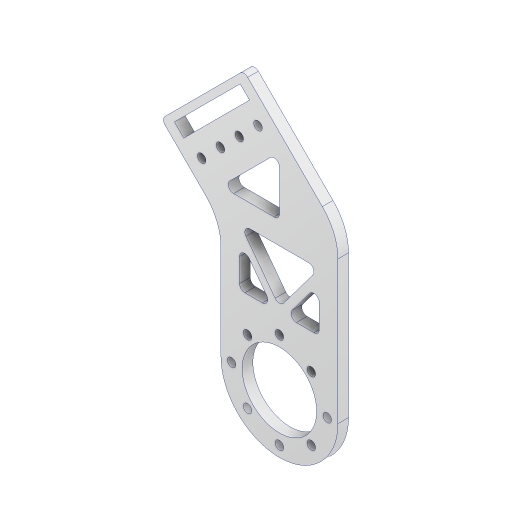
# Autodesk Inventor part: 조인트3힌지사이드_4T
Saved by Autodesk Inventor 2023.2 (Build 272271000, 271)
## iProperties
Created: 2022-01-19
Part Number: 조인트3힌지사이드_4T
Material: 알루미늄 6061
Document SubType Name: Modeling
Designer: BAEK
Density: 2.7 g/cm^3
Appearance: 알루미늄 - 평지
Mass: 34.6607 g
Surface Area: 93.0262 cm^2
Volume: 12.8373 cm^3
Author: BAEK
Autodesk Inventor part; units mm, degrees
ref_plane "YZ Plane" through (0, 0, 0) normal (1, 0, 0) x (0, 1, 0)
ref_plane "XZ Plane" through (0, 0, 0) normal (0, 1, 0) x (-1, 0, 0)
ref_plane "XY Plane" through (0, 0, 0) normal (0, 0, 1) x (1, 0, 0)
sketch "스케치1" plane through (0, 0, 0) normal (0, 0, 1) x (1, 0, 0)
  circle A0 centre (0, 0) radius 22
  line L0 (0, 0) -> (0, 18)
  line L1 (-0.15, -20.7995) -> (-0.15, -19.593)
  arc A1 (-0.15, -16.407) -> (-0.15, -19.593) centre (0, -18) ccw
  line L2 (-0.15, -16.407) -> (-0.15, -12.9991)
  arc A2 (0.15, -12.9991) -> (-0.15, -12.9991) centre (0, 0) ccw
  line L3 (0.15, -16.407) -> (0.15, -12.9991)
  arc A3 (0.15, -19.593) -> (0.15, -16.407) centre (0, -18) ccw
  line L4 (0.15, -20.7995) -> (0.15, -19.593)
  circle A4 centre (12, 12) radius 1.6
  circle A5 centre (-18, 0) radius 1.6
  circle A6 centre (-12, 12) radius 1.6
  circle A7 centre (-12, -12) radius 1.6
  circle A8 centre (18, 0) radius 1.6
  circle A9 centre (12, -12) radius 1.6
  circle A10 centre (0, 18) radius 1.6
  circle A11 centre (0, 0) radius 12.5
  circle A12 centre (0, -18) radius 1.6
  point P0 (0.15, -19.593)
  dimension "d0" = 44
  dimension "d1" = 18
  constraints: 13 centre point, 10 end point, 6 point on circle, 2 coincident, 1 concentric, 1 vertical
  measures "d0" diameter of A0
  measures "d1" distance of L0.start L0.end
extrude "돌출1" add sketch "스케치1" along normal blind 4 contours A0 | A2 L3 A12 L2 | A10 | A11 | A3 A12 A1 | A4 | A5 | A6 | A7 | A8 | A9
sketch "스케치2" plane through (0, 0, 4) normal (0, 0, 1) x (1, 0, 0)
  circle A0 centre (0, 0) radius 22 projected
  circle A1 centre (0, 0) radius 22 projected
  line L0 (0, -22) -> (0, 58)
  line L1 (22, 0) -> (22, 53.7157)
  line L2 (16.1421, 67.8579) -> (-6.2843, 90.2843)
  line L3 (22, 62) -> (53.7157, 62) construction
  line L4 (-6.2843, 90.2843) -> (-37.397, 59.1716)
  line L5 (-22, 0) -> (-22, 35.4903)
  line L6 (-27.8579, 49.6325) -> (-37.397, 59.1716)
  arc A2 (-22, 35.4903) -> (-27.8579, 49.6325) centre (-42, 35.4903) ccw
  arc A3 (22, 53.7157) -> (16.1421, 67.8579) centre (2, 53.7157) ccw
  point P0 (-22, 43.7746)
  dimension "d9" = 80
  dimension "d46" = 62
  dimension "d48" = 135
  dimension "d50" = 40
  dimension "d57" = 20
  dimension "d92" = 44
  constraints: 14 end point, 8 tangent, 7 point on circle, 4 point on line, 3 vertical, 2 centre point, 2 perpendicular, 1 equal length, 1 equal radius, 1 horizontal
  measures "d9" distance of L0.start L0.end
  measures "d46" distance of L1.start L3.start
  measures "d48" angle of L3 L2
  measures "d50" distance of L3.start L2.end
  measures "d57" radius of A2
  measures "d92" distance of L2.end L4.end
sketch "스케치4" plane through (0, 0, 4) normal (0, 0, 1) x (1, 0, 0)
  circle A0 centre (0, 0) radius 14
  dimension "d32" = 28
  constraints: 1 centre point, 1 coincident
  measures "d32" diameter of A0
extrude "돌출4" cut sketch "스케치4" against normal blind 4
sketch "스케치5" plane through (0, 0, 4) normal (0, 0, 1) x (1, 0, 0)
  line L0 (-0.0007, 55) -> (-0.0007, 47)
  line L1 (-0.0007, 47) -> (10.9993, 47)
  line L2 (-0.0007, 47) -> (-11.0007, 47)
  line L3 (-0.0007, 47) -> (-0.0007, 27)
  line L4 (-12.6007, 43.8) -> (-1.6007, 29.1333)
  line L5 (12.5993, 43.8) -> (1.5993, 29.1333)
  line L6 (11.3993, 37.2) -> (4.7993, 28.4)
  line L7 (6.3993, 25.2) -> (12.9993, 25.2)
  line L8 (14.9993, 27.2) -> (14.9993, 36)
  arc A0 (-11.0007, 47) -> (-12.6007, 43.8) centre (-11.0007, 45) ccw
  arc A1 (-1.6007, 29.1333) -> (1.5993, 29.1333) centre (-0.0007, 30.3333) ccw
  arc A2 (12.5993, 43.8) -> (10.9993, 47) centre (10.9993, 45) ccw
  arc A3 (14.9993, 36) -> (11.3993, 37.2) centre (12.9993, 36) ccw
  arc A4 (12.9993, 25.2) -> (14.9993, 27.2) centre (12.9993, 27.2) ccw
  arc A5 (4.7993, 28.4) -> (6.3993, 25.2) centre (6.3993, 27.2) ccw
  line L9 (-11.4007, 37.2) -> (-4.8007, 28.4)
  line L10 (-6.4007, 25.2) -> (-13.0007, 25.2)
  line L11 (-15.0007, 27.2) -> (-15.0007, 36)
  arc A6 (-11.4007, 37.2) -> (-15.0007, 36) centre (-13.0007, 36) ccw
  arc A7 (-15.0007, 27.2) -> (-13.0007, 25.2) centre (-13.0007, 27.2) ccw
  arc A8 (-6.4007, 25.2) -> (-4.8007, 28.4) centre (-6.4007, 27.2) ccw
  point P0 (0, 0)
  point P1 (14.9993, 47)
  point P2 (-15.0007, 47)
  point P3 (14.9993, 42)
  dimension "d35" = 8
  dimension "d36" = 15
  dimension "d37" = 15
  dimension "d38" = 20
  dimension "d39" = 5
  dimension "d41" = 2
  constraints: 24 end point, 18 point on circle, 12 tangent, 9 centre point, 9 symmetric about line, 8 point on line, 5 equal radius, 3 horizontal, 2 vertical, 1 parallel, 1 perpendicular, 3 other
  measures "d35" distance of L0.start L0.end
  measures "d36" distance of L0.end point (14.999, 47)
  measures "d37" distance of L0.end point (-15.001, 47)
  measures "d38" distance of L0.end L3.end
  measures "d39" distance of point (14.999, 47) point (14.999, 42)
  measures "d41" radius of A0
extrude "돌출7" add sketch "스케치2" against normal blind 4 contours L5 A2 L6 L4 L2 A3 L1 A0
extrude "돌출8" cut sketch "스케치5" against normal blind 4
extrude "돌출9" cut sketch "스케치1" along normal blind 4 contours A10 | A3 A12 A1 | A4 | A5 | A6 | A7 | A8 | A9
sketch "스케치9" plane through (0, 0, 4) normal (0, 0, 1) x (1, 0, 0)
  circle A0 centre (-12, 12) radius 1.6 projected
  circle A1 centre (12, -12) radius 1.6 projected
  circle A2 centre (0, -18) radius 1.6 projected
  circle A3 centre (0, 18) radius 1.6 projected
  circle A4 centre (-18, 0) radius 1.6 projected
  circle A5 centre (18, 0) radius 1.6 projected
  circle A6 centre (-12, -12) radius 1.6 projected
  circle A7 centre (12, 12) radius 1.6 projected
  line L0 (4.7993, 28.4) -> (11.3993, 37.2) projected
  arc A8 (14.9993, 36) -> (11.3993, 37.2) centre (12.9993, 36) ccw projected
  line L1 (14.9993, 36) -> (14.9993, 27.2) projected
  arc A9 (12.9993, 25.2) -> (14.9993, 27.2) centre (12.9993, 27.2) ccw projected
  line L2 (12.9993, 25.2) -> (6.3993, 25.2) projected
  arc A10 (4.7993, 28.4) -> (6.3993, 25.2) centre (6.3993, 27.2) ccw projected
  arc A11 (-6.4007, 25.2) -> (-4.8007, 28.4) centre (-6.4007, 27.2) ccw projected
  line L3 (-6.4007, 25.2) -> (-13.0007, 25.2) projected
  arc A12 (-15.0007, 27.2) -> (-13.0007, 25.2) centre (-13.0007, 27.2) ccw projected
  line L4 (-15.0007, 27.2) -> (-15.0007, 36) projected
  arc A13 (-11.4007, 37.2) -> (-15.0007, 36) centre (-13.0007, 36) ccw projected
  line L5 (-11.4007, 37.2) -> (-4.8007, 28.4) projected
  line L6 (12.5993, 43.8) -> (1.5993, 29.1333) projected
  arc A14 (-1.6007, 29.1333) -> (1.5993, 29.1333) centre (-0.0007, 30.3333) ccw projected
  line L7 (-1.6007, 29.1333) -> (-12.6007, 43.8) projected
  arc A15 (-11.0007, 47) -> (-12.6007, 43.8) centre (-11.0007, 45) ccw projected
  line L8 (-11.0007, 47) -> (10.9993, 47) projected
  arc A16 (12.5993, 43.8) -> (10.9993, 47) centre (10.9993, 45) ccw projected
  circle A17 centre (0, 0) radius 14 projected
  arc A18 (-22, 0) -> (22, 0) centre (0, 0) ccw projected
  line L9 (22, 0) -> (22, 53.7157) projected
  arc A19 (22, 53.7157) -> (16.1421, 67.8579) centre (2, 53.7157) ccw projected
  line L10 (16.1421, 67.8579) -> (-6.2843, 90.2843) projected
  line L11 (-6.2843, 90.2843) -> (-37.397, 59.1716) projected
  line L12 (-37.397, 59.1716) -> (-27.8579, 49.6325) projected
  arc A20 (-22, 35.4903) -> (-27.8579, 49.6325) centre (-42, 35.4903) ccw projected
  line L13 (-22, 35.4903) -> (-22, 0) projected
  circle A21 centre (-29.2652, 60.9393) radius 1.6
  circle A22 centre (-22.1942, 68.0104) radius 1.6
  circle A23 centre (-15.1231, 75.0815) radius 1.6
  circle A24 centre (-8.052, 82.1525) radius 1.6
  dimension "d73" = 3.2
  dimension "d74" = 3.2
  dimension "d76" = 3.2
  dimension "d77" = 3.2
  dimension "d78" = 4.5
  dimension "d79" = 4.5
  dimension "d81" = 4.5
  dimension "d82" = 4.5
  dimension "d83" = 10
  dimension "d85" = 10
  dimension "d88" = 7
  dimension "d91" = 7
  constraints: 4 centre point
  measures "d73" diameter of A21
  measures "d74" diameter of A22
  measures "d76" diameter of A23
  measures "d77" diameter of A24
  measures "d78" distance from line of L11 A21.centre
  measures "d79" distance from line of L11 A22.centre
  measures "d81" distance from line of L11 A23.centre
  measures "d82" distance from line of L11 A24.centre
  measures "d83" distance of A22.centre A21.centre
  measures "d85" distance of A23.centre A24.centre
  measures "d88" distance from line of L12 A21.centre
  measures "d91" distance from line of L10 A24.centre
extrude "돌출10" cut sketch "스케치9" against normal blind 10 contours A21 | A22 | A23 | A24
sketch "스케치10" plane through (0, 0, 4) normal (0, 0, 1) x (1, 0, 0)
  circle A0 centre (-15.1231, 75.0815) radius 1.6 projected
  circle A1 centre (-22.1942, 68.0104) radius 1.6 projected
  circle A2 centre (-8.052, 82.1525) radius 1.6 projected
  circle A3 centre (-29.2652, 60.9393) radius 1.6 projected
  circle A4 centre (-12, 12) radius 1.6 projected
  circle A5 centre (12, -12) radius 1.6 projected
  circle A6 centre (0, -18) radius 1.6 projected
  circle A7 centre (0, 18) radius 1.6 projected
  circle A8 centre (-18, 0) radius 1.6 projected
  circle A9 centre (18, 0) radius 1.6 projected
  circle A10 centre (-12, -12) radius 1.6 projected
  circle A11 centre (12, 12) radius 1.6 projected
  line L0 (4.7993, 28.4) -> (11.3993, 37.2) projected
  arc A12 (14.9993, 36) -> (11.3993, 37.2) centre (12.9993, 36) ccw projected
  line L1 (14.9993, 36) -> (14.9993, 27.2) projected
  arc A13 (12.9993, 25.2) -> (14.9993, 27.2) centre (12.9993, 27.2) ccw projected
  line L2 (12.9993, 25.2) -> (6.3993, 25.2) projected
  arc A14 (4.7993, 28.4) -> (6.3993, 25.2) centre (6.3993, 27.2) ccw projected
  arc A15 (-6.4007, 25.2) -> (-4.8007, 28.4) centre (-6.4007, 27.2) ccw projected
  line L3 (-6.4007, 25.2) -> (-13.0007, 25.2) projected
  arc A16 (-15.0007, 27.2) -> (-13.0007, 25.2) centre (-13.0007, 27.2) ccw projected
  line L4 (-15.0007, 27.2) -> (-15.0007, 36) projected
  arc A17 (-11.4007, 37.2) -> (-15.0007, 36) centre (-13.0007, 36) ccw projected
  line L5 (-11.4007, 37.2) -> (-4.8007, 28.4) projected
  line L6 (12.5993, 43.8) -> (1.5993, 29.1333) projected
  arc A18 (-1.6007, 29.1333) -> (1.5993, 29.1333) centre (-0.0007, 30.3333) ccw projected
  line L7 (-1.6007, 29.1333) -> (-12.6007, 43.8) projected
  arc A19 (-11.0007, 47) -> (-12.6007, 43.8) centre (-11.0007, 45) ccw projected
  line L8 (-11.0007, 47) -> (10.9993, 47) projected
  arc A20 (12.5993, 43.8) -> (10.9993, 47) centre (10.9993, 45) ccw projected
  circle A21 centre (0, 0) radius 14 projected
  arc A22 (-22, 0) -> (22, 0) centre (0, 0) ccw projected
  line L9 (22, 0) -> (22, 53.7157) projected
  arc A23 (22, 53.7157) -> (16.1421, 67.8579) centre (2, 53.7157) ccw projected
  line L10 (16.1421, 67.8579) -> (-6.2843, 90.2843) projected
  line L11 (-6.2843, 90.2843) -> (-37.397, 59.1716) projected
  line L12 (-37.397, 59.1716) -> (-27.8579, 49.6325) projected
  arc A24 (-22, 35.4903) -> (-27.8579, 49.6325) centre (-42, 35.4903) ccw projected
  line L13 (-22, 35.4903) -> (-22, 0) projected
  line L14 (-6.2843, 90.2843) -> (16.1421, 67.8579) projected
  line L15 (-6.2843, 90.2843) -> (-13.3553, 97.3553)
  line L16 (-13.3553, 97.3553) -> (-44.468, 66.2426)
  line L17 (-44.468, 66.2426) -> (-37.397, 59.1716)
  line L18 (-14.7696, 92.4056) -> (-39.5183, 67.6569)
  line L19 (-6.2843, 90.2843) -> (-37.397, 59.1716) projected
  line L20 (-39.5183, 67.6569) -> (-35.9828, 64.1213)
  line L21 (-35.9828, 64.1213) -> (-11.234, 88.8701)
  line L22 (-11.234, 88.8701) -> (-14.7696, 92.4056)
  point P0 (-37.397, 59.1716)
  dimension "d93" = 10
  dimension "d95" = 5
  dimension "d96" = 35
  dimension "d97" = 2.5
  dimension "d99" = 4.5
  constraints: 14 end point, 4 perpendicular, 2 parallel, 1 collinear
  measures "d93" distance of L10.end L15.end
  measures "d95" distance of L21.end L18.start
  measures "d96" distance of L18.start L18.end
  measures "d97" distance between parallel lines of L16 L18
  measures "d99" distance between parallel lines of L15 L22
extrude "돌출11" add sketch "스케치10" against normal blind 4 contours L17 L16 L15 L11
fillet "모깎기1" radius 2 2 edges at (-13.3553, 97.3553, 2) (-44.468, 66.2426, 2)
sketch "스케치11" plane through (0, 0, 4) normal (0, 0, 1) x (1, 0, 0)
  arc A0 (-43.0538, 67.6569) -> (-43.0538, 64.8284) centre (-41.6396, 66.2426) ccw projected
  line L0 (-43.0538, 64.8284) -> (-27.8579, 49.6325) projected
  arc A1 (-22, 35.4903) -> (-27.8579, 49.6325) centre (-42, 35.4903) ccw projected
  line L1 (-22, 35.4903) -> (-22, 0) projected
  arc A2 (-22, 0) -> (22, 0) centre (0, 0) ccw projected
  line L2 (22, 0) -> (22, 53.7157) projected
  arc A3 (22, 53.7157) -> (16.1421, 67.8579) centre (2, 53.7157) ccw projected
  line L3 (16.1421, 67.8579) -> (-11.9411, 95.9411) projected
  arc A4 (-11.9411, 95.9411) -> (-14.7696, 95.9411) centre (-13.3553, 94.5269) ccw projected
  line L4 (-14.7696, 95.9411) -> (-43.0538, 67.6569) projected
  line L5 (-35.9828, 64.1213) -> (-39.5183, 67.6569) projected
  line L6 (-39.5183, 67.6569) -> (-14.7696, 92.4056) projected
  line L7 (-14.7696, 92.4056) -> (-11.234, 88.8701) projected
  line L8 (-11.234, 88.8701) -> (-35.9828, 64.1213) projected
  circle A5 centre (-15.1231, 75.0815) radius 1.6 projected
  circle A6 centre (-22.1942, 68.0104) radius 1.6 projected
  circle A7 centre (-8.052, 82.1525) radius 1.6 projected
  circle A8 centre (-29.2652, 60.9393) radius 1.6 projected
  circle A9 centre (-12, 12) radius 1.6 projected
  circle A10 centre (12, -12) radius 1.6 projected
  circle A11 centre (0, -18) radius 1.6 projected
  circle A12 centre (0, 18) radius 1.6 projected
  circle A13 centre (-18, 0) radius 1.6 projected
  circle A14 centre (18, 0) radius 1.6 projected
  circle A15 centre (-12, -12) radius 1.6 projected
  circle A16 centre (12, 12) radius 1.6 projected
  arc A17 (4.7993, 28.4) -> (6.3993, 25.2) centre (6.3993, 27.2) ccw projected
  line L9 (4.7993, 28.4) -> (11.3993, 37.2) projected
  arc A18 (14.9993, 36) -> (11.3993, 37.2) centre (12.9993, 36) ccw projected
  line L10 (14.9993, 36) -> (14.9993, 27.2) projected
  arc A19 (12.9993, 25.2) -> (14.9993, 27.2) centre (12.9993, 27.2) ccw projected
  line L11 (12.9993, 25.2) -> (6.3993, 25.2) projected
  arc A20 (-6.4007, 25.2) -> (-4.8007, 28.4) centre (-6.4007, 27.2) ccw projected
  line L12 (-6.4007, 25.2) -> (-13.0007, 25.2) projected
  arc A21 (-15.0007, 27.2) -> (-13.0007, 25.2) centre (-13.0007, 27.2) ccw projected
  line L13 (-15.0007, 27.2) -> (-15.0007, 36) projected
  arc A22 (-11.4007, 37.2) -> (-15.0007, 36) centre (-13.0007, 36) ccw projected
  line L14 (-11.4007, 37.2) -> (-4.8007, 28.4) projected
  line L15 (-11.0007, 47) -> (10.9993, 47) projected
  arc A23 (12.5993, 43.8) -> (10.9993, 47) centre (10.9993, 45) ccw projected
  line L16 (12.5993, 43.8) -> (1.5993, 29.1333) projected
  arc A24 (-1.6007, 29.1333) -> (1.5993, 29.1333) centre (-0.0007, 30.3333) ccw projected
  line L17 (-1.6007, 29.1333) -> (-12.6007, 43.8) projected
  arc A25 (-11.0007, 47) -> (-12.6007, 43.8) centre (-11.0007, 45) ccw projected
  circle A26 centre (0, 0) radius 14 projected
  arc A27 (46.1675, 71.3111) -> (47.7675, 68.1111) centre (47.7675, 70.1111) ccw
  line L18 (46.1675, 71.3111) -> (52.7675, 80.1111)
  arc A28 (56.3675, 78.9111) -> (52.7675, 80.1111) centre (54.3675, 78.9111) ccw
  line L19 (56.3675, 78.9111) -> (56.3675, 70.1111)
  arc A29 (54.3675, 68.1111) -> (56.3675, 70.1111) centre (54.3675, 70.1111) ccw
  line L20 (54.3675, 68.1111) -> (47.7675, 68.1111)
  arc A30 (34.9675, 68.1111) -> (36.5675, 71.3111) centre (34.9675, 70.1111) ccw
  line L21 (34.9675, 68.1111) -> (28.3675, 68.1111)
  arc A31 (26.3675, 70.1111) -> (28.3675, 68.1111) centre (28.3675, 70.1111) ccw
  line L22 (26.3675, 70.1111) -> (26.3675, 78.9111)
  arc A32 (29.9675, 80.1111) -> (26.3675, 78.9111) centre (28.3675, 78.9111) ccw
  line L23 (29.9675, 80.1111) -> (36.5675, 71.3111)
  line L24 (30.3675, 89.9111) -> (52.3675, 89.9111)
  arc A33 (53.9675, 86.7111) -> (52.3675, 89.9111) centre (52.3675, 87.9111) ccw
  line L25 (53.9675, 86.7111) -> (42.9675, 72.0445)
  arc A34 (39.7675, 72.0445) -> (42.9675, 72.0445) centre (41.3675, 73.2445) ccw
  line L26 (39.7675, 72.0445) -> (28.7675, 86.7111)
  arc A35 (30.3675, 89.9111) -> (28.7675, 86.7111) centre (30.3675, 87.9111) ccw
  line L27 (-43.0538, 64.8284) -> (-27.8579, 49.6325) projected
  line L28 (16.1421, 67.8579) -> (-11.9411, 95.9411) projected
  line L29 (-11.0007, 47) -> (10.9993, 47) projected
  line L30 (-0.0007, 47) -> (-0.0007, 52)
  line L31 (22, 53.7157) -> (22, 0) projected
  arc A36 (-22, 35.4903) -> (-27.8579, 49.6325) centre (-42, 35.4903) ccw projected
  line L32 (-27.8579, 49.6325) -> (3.2548, 80.7452)
  line L33 (-22.0662, 55.4241) -> (-0.0007, 55.4241)
  line L34 (-0.0007, 55.4241) -> (-0.0007, 77.4896)
  dimension "d103" = 5
  dimension "d104" = 22.0655
  constraints: 26 end point, 18 point on circle, 9 centre point, 3 point on line, 2 perpendicular, 1 horizontal, 1 midpoint, 1 vertical
  measures "d103" distance of L30.start L30.end
  measures "d104" distance of L33.end L34.end
extrude "돌출12" cut sketch "스케치11" against normal blind 10 contours L32 L34 L33
fillet "모깎기2" radius 2 3 edges at (-22.0662, 55.4241, 2) (-0.0007, 77.4896, 2) (-0.0007, 55.4241, 2)
